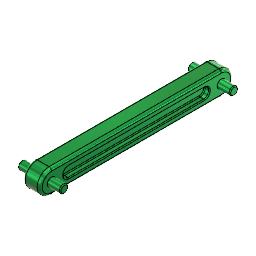
2nd link (Autodesk Fusion 360 design; units mm, degrees)
Autodesk Fusion 360 part; units mm, degrees
sketch "Sketch3" plane through (0, 0, 0) normal (1, 0, 0) x (0, 0, -1)
  circle A0 centre (0, 650) radius 25
  line L0 (0, 720) -> (-1000, 720)
  arc A1 (-1000, 720) -> (-1000, 580) centre (-1000, 650) ccw
  line L1 (-1000, 580) -> (0, 580)
  arc A2 (0, 580) -> (0, 720) centre (0, 650) ccw
  line L2 (0, 650) -> (-1000, 650) construction
  arc A3 (75, 650) -> (-75, 650) centre (0, 650) ccw
  dimension "d1" = 1000
  dimension "d2" = 70
  constraint tangent L0 A1
  constraint tangent A1 L1
  constraint parallel L0 L1
  constraint tangent L1 A2
  constraint tangent L0 A2
  constraint horizontal L2
  constraint coincident A0.centre A2.centre
  measures "d1" distance of A0.centre A1.centre
  measures "d2" radius of A2
extrude "Extrude1" add sketch "Sketch3" along normal mid plane 100 contours A0 | L0 A1 L1 A2
sketch "Sketch1" plane through (50, 0, 0) normal (1, 0, 0) x (0, 0, -1)
  arc A0 (0, 580) -> (0, 720) centre (0, 650) ccw
  line L0 (0, 720) -> (-1000, 720)
  arc A1 (-1000, 720) -> (-1000, 580) centre (-1000, 650) ccw
  line L1 (-1000, 580) -> (0, 580)
  circle A2 centre (-1000, 650) radius 25
  circle A3 centre (0, 650) radius 25
  dimension "d39" = 50
  dimension "d40" = 50
  constraint concentric A1 A2
  constraint concentric A0 A3
  measures "d39" diameter of A3
  measures "d40" diameter of A2
extrude "Extrude2" add sketch "Sketch1" along normal blind 75 contours A2 | A3
mirror "Mirror1" about plane through (0, 0, 0) normal (1, 0, 0) of "Extrude2"
chamfer "Chamfer1" distance 5 angle 45 4 edges at (125, 640.9596, 1023.3082) (125, 640.9596, 23.3082) (-125, 640.9596, 1023.3082) (-125, 640.9596, 23.3082)
fillet "Fillet1" radius 15 8 edges at (50, 580, 500) (50, 650, -70) (50, 720, 500) (50, 650, 1070) (-50, 580, 500) (-50, 650, 1070) (-50, 720, 500) (-50, 650, -70)
sketch "Sketch2" plane through (-50, 0, 0) normal (-1, 0, 0) x (0, 0, 1)
  circle A0 centre (1000, 650) radius 25
  circle A1 centre (0, 650) radius 25
  line L0 (0, 595) -> (1000, 595)
  arc A2 (1000, 595) -> (1000, 705) centre (1000, 650) ccw
  line L1 (1000, 705) -> (0, 705)
  arc A3 (0, 705) -> (0, 595) centre (0, 650) ccw
  line L2 (100, 620) -> (900, 620)
  arc A4 (900, 620) -> (900, 680) centre (900, 650) ccw
  line L3 (900, 680) -> (100, 680)
  arc A5 (100, 680) -> (100, 620) centre (100, 650) ccw
  line L4 (100, 650) -> (900, 650) construction
  circle A6 centre (1000, 650) radius 20
  circle A7 centre (0, 650) radius 20
  dimension "d46" = 100
  dimension "d47" = 100
  dimension "d48" = 30
  constraint tangent L2 A4
  constraint tangent A4 L3
  constraint parallel L2 L3
  constraint tangent L3 A5
  constraint tangent L2 A5
  constraint parallel L0 L4
  constraint horizontal A1.centre A5.centre
  measures "d46" distance of A5.centre A1.centre
  measures "d47" distance of A0.centre A4.centre
  measures "d48" radius of A4
extrude "Extrude3" cut sketch "Sketch2" against normal blind 30 contours L2 A4 L3 A5
mirror "Mirror2" about plane through (0, 0, 0) normal (1, 0, 0) of "Extrude3"
fillet "Fillet2" radius 5 16 edges at (50, 680, 500) (50, 650, 70) (50, 620, 500) (50, 650, 930) (20, 680, 500) (20, 650, 930) (20, 620, 500) (20, 650, 70) (-20, 680, 500) (-20, 650, 930) (-20, 620, 500) (-20, 650, 70) (-50, 680, 500) (-50, 650, 930) (-50, 620, 500) (-50, 650, 70)
